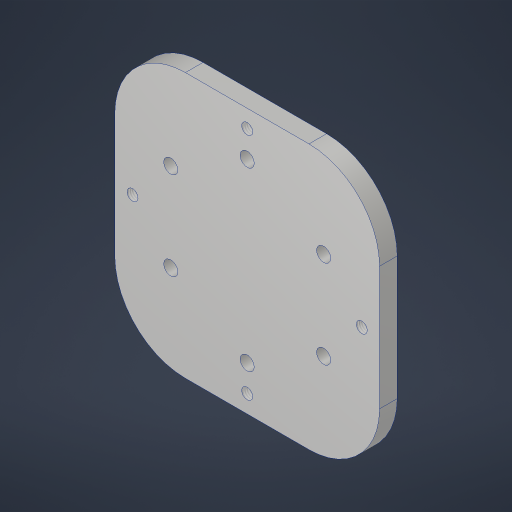
# Autodesk Inventor part: GP6-004
Saved by Autodesk Inventor 2023.4 (Build 274418000, 418)
## iProperties
RuleStatus: InUse
Created: 2025-02-23
Part Number: GP6-004
Material: Aluminum 6061
Document SubType Name: Modeling
Designer: brand
Mass: 132.735 g
Surface Area: 177.419 cm^2
Volume: 49.1612 cm^3
Density: 2.7 g/cm^3
Appearance: Aluminum - Flat
AfterDocNew0: SHOW
AfterDocOpen0: SHOW
Author: brand
Autodesk Inventor part; units mm, degrees
ref_plane "YZ Plane" through (0, 0, 0) normal (1, 0, 0) x (0, 1, 0)
ref_plane "XZ Plane" through (0, 0, 0) normal (0, 1, 0) x (-1, 0, 0)
ref_plane "XY Plane" through (0, 0, 0) normal (0, 0, 1) x (1, 0, 0)
sketch "Sketch1" plane through (0, 0, 0) normal (0, 0, 1) x (1, 0, 0)
  line L0 (-47.625, -47.625) -> (47.625, -47.625)
  line L1 (47.625, -47.625) -> (47.625, 47.625)
  line L2 (47.625, 47.625) -> (-47.625, 47.625)
  line L3 (-47.625, 47.625) -> (-47.625, -47.625)
  line L4 (-47.625, -47.625) -> (47.625, 47.625) construction
  line L5 (47.625, -47.625) -> (-47.625, 47.625) construction
  point P0 (0, 0)
  dimension "width" = 95.25
  dimension "length" = 95.25
  constraints: 12 end point, 2 midpoint, 2 parallel, 1 horizontal, 1 perpendicular
  measures "width" distance of L2.end L1.end
  measures "length" distance of L0.end L1.end
extrude "Extrusion1" add sketch "Sketch1" along normal mid plane 6.35
sketch "Sketch2" plane through (0, 0, 3.175) normal (0, 0, 1) x (1, 0, 0)
  circle A0 centre (0, 0) radius 35
  circle A1 centre (0, 0) radius 60 construction
  circle A2 centre (0, 0) radius 47.5
  line L0 (0, 35) -> (0, 60) construction
  line L1 (0, 47.5) -> (0, 35) construction
  point P0 (0, 41.25)
  point P1 (-41.25, 0)
  point P2 (0, -41.25)
  point P3 (41.25, 0)
  dimension "d4" = 70
  dimension "d5" = 120
  dimension "d8" = 360
  constraints: 4 end point, 4 vertical alignment, 3 coincident, 2 midpoint, 2 vertical, 11 other
hole "Hole1" at (0, 41.25, 3.175) at (-41.25, 0, 3.175) at (0, -41.25, 3.175) at (41.25, 0, 3.175) direction (0, 0, -1) diameter 3.9624 end through all thread size "10-32 UNF" class "2B" standard "ANSI Unified Screw Threads"
sketch "Sketch3" plane through (0, 0, 3.175) normal (0, 0, 1) x (1, 0, 0)
  circle A0 centre (0, 0) radius 31.75 construction
  point P0 (0, 31.75)
  point P1 (-27.4963, 15.875)
  point P2 (-27.4963, -15.875)
  point P3 (0, -31.75)
  point P4 (27.4963, -15.875)
  point P5 (27.4963, 15.875)
  dimension "d17" = 63.5
  dimension "d20" = 360
  constraints: 2 vertical alignment, 1 coincident, 9 other
hole "Hole2" at (0, 31.75, 3.175) at (-27.4963, 15.875, 3.175) at (-27.4963, -15.875, 3.175) at (0, -31.75, 3.175) at (27.4963, -15.875, 3.175) at (27.4963, 15.875, 3.175) direction (0, 0, -1) diameter 5.1054 end through all clearance for "Hex Machine Screw" size "#10" standard "Ansi Unified Screw Threads"
fillet "Fillet1" radius 25.4 4 edges at (47.625, 47.625, 0) (-47.625, 47.625, 0) (-47.625, -47.625, 0) (47.625, -47.625, 0)
body "Solid1"
